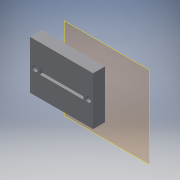
# Autodesk Inventor part: Breadboard
Saved by Autodesk Inventor 2016 (Build 200138000, 138)
## iProperties
Created: 2017-06-15
Part Number: Breadboard
Material: Generic
Document SubType Name: Modeling
Designer: Owner
Density: 1 g/cm^3
Appearance: Default
Author: Owner
Autodesk Inventor part; units mm, degrees
ref_plane "YZ Plane" through (0, 0, 0) normal (1, 0, 0) x (0, 1, 0)
ref_plane "XZ Plane" through (0, 0, 0) normal (0, 1, 0) x (-1, 0, 0)
ref_plane "XY Plane" through (0, 0, 0) normal (0, 0, 1) x (1, 0, 0)
ref_plane "Work Plane1" through (0, 0, 0) normal (0, 0, 1) x (1, 0, 0)
sketch "Sketch1" plane through (0, 0, 0) normal (0, 0, 1) x (1, 0, 0)
  line L0 (-75.8806, 15.6994) -> (-120.8806, 15.6994)
  line L1 (-120.8806, 15.6994) -> (-120.8806, -18.8006)
  line L2 (-120.8806, -18.8006) -> (-75.8806, -18.8006)
  line L3 (-75.8806, -18.8006) -> (-75.8806, 15.6994)
  point P0 (0, 0)
  dimension "d0" = 34.5
  dimension "d1" = 45
  constraints: 8 end point, 2 parallel, 1 horizontal, 1 perpendicular
  measures "d0" distance of L2.end L0.start
  measures "d1" distance of L1.end L2.end
extrude "Extrusion1" add sketch "Sketch1" along normal blind 8.5
sketch "Sketch2" plane through (0, 0, 8.5) normal (0, 0, 1) x (1, 0, 0)
  line L0 (-120.8806, 15.6994) -> (-120.8806, -18.8006) projected
  line L1 (-120.8806, -1.5506) -> (-113.8806, -1.5506)
  line L2 (-113.8806, -1.5506) -> (-82.8806, -1.5506)
  line L3 (-82.8806, -1.5506) -> (-82.8806, -4.0506)
  line L4 (-82.8806, -1.5506) -> (-82.8806, 0.9494)
  line L5 (-82.8806, -4.0506) -> (-113.8806, -4.0506)
  line L6 (-113.8806, -4.0506) -> (-113.8806, 0)
  line L7 (-113.8806, 0) -> (-82.8806, 0)
  line L8 (-82.8806, 0) -> (-82.8806, -4.0506)
  line L9 (-82.8806, -4.0506) -> (-113.8806, -4.0506)
  line L10 (-113.8806, -4.0506) -> (-113.8806, 0)
  line L11 (-113.8806, 0) -> (-82.8806, 0)
  line L12 (-82.8806, 0) -> (-82.8806, -4.0506)
  point P0 (0, 0)
  dimension "d4" = 7
  dimension "d5" = 31
  dimension "d6" = 2.5
  dimension "d7" = 2.5
  constraints: 24 end point, 4 parallel, 3 horizontal, 2 coincident, 2 perpendicular, 2 vertical, 1 midpoint, 1 point on line
  measures "d4" distance of L1.start L1.end
  measures "d5" distance of L1.end L2.end
  measures "d6" distance of L2.end L3.end
  measures "d7" distance of L2.end L4.end
extrude "Extrusion2" cut sketch "Sketch2" against normal blind 2
sketch "Sketch3" plane through (0, 0, 8.5) normal (0, 0, 1) x (1, 0, 0)
  line L0 (-82.8806, 0) -> (-82.8806, -4.0506) projected
  line L1 (-113.8806, 0) -> (-82.8806, 0) projected
  line L2 (-113.8806, -4.0506) -> (-113.8806, 0) projected
  line L3 (-82.8806, -4.0506) -> (-113.8806, -4.0506) projected
  line L4 (-75.8806, -18.8006) -> (-75.8806, 15.6994) projected
  line L5 (-82.8806, -2.0253) -> (-79.3754, -2.0253)
  line L6 (-113.8806, -2.0253) -> (-117.3858, -2.0253)
  circle A0 centre (-117.3858, -2.0253) radius 2.0253
  circle A1 centre (-79.3754, -2.0253) radius 2.0253
  point P0 (0, 0)
  dimension "d11" = 3.5052
  dimension "d12" = 3.5052
  constraints: 4 end point, 2 centre point, 2 coincident, 2 horizontal, 2 midpoint
  measures "d11" distance of L5.start L5.end
  measures "d12" distance of L6.start L6.end
extrude "Extrusion3" cut sketch "Sketch3" against normal blind 2 contours A1 | A0
body "Solid1"
